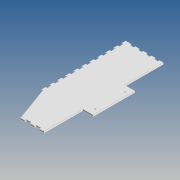
# Autodesk Inventor part: KB33-046-004-008 - Центральная правая боковая пластина
Saved by Autodesk Inventor 2020 (Build 240168000, 168)
## iProperties
Created: 2021-06-25
Part Number: KB33-046-004-008 - Центральная правая боковая пластина
Material: Типовые
Document SubType Name: Modeling
Designer: Петров Иван
Density: 1 g/cm^3
Appearance: По умолчанию
Mass: 112.867 g
Surface Area: 603.849 cm^2
Volume: 112.867 cm^3
Author: Петров Иван
Autodesk Inventor part; units mm, degrees
ref_plane "YZ Plane" through (0, 0, 0) normal (1, 0, 0) x (0, 1, 0)
ref_plane "XZ Plane" through (0, 0, 0) normal (0, 1, 0) x (-1, 0, 0)
ref_plane "XY Plane" through (0, 0, 0) normal (0, 0, 1) x (1, 0, 0)
sketch "Эскиз1" plane through (2.236, 0, -46.8876) normal (0, 1, 0) x (-1, 0, 0)
  line L0 (-10.528, 98.8876) -> (15, 98.8876)
  line L1 (15, 98.8876) -> (15, -5.1124)
  line L2 (15, -5.1124) -> (-10.528, -5.1124)
  line L3 (-10.528, -5.1124) -> (-10.528, 98.8876)
  point P0 (0, 0)
  dimension "d0" = 25.528
  dimension "d1" = 104
  constraints: 8 end point, 2 parallel, 1 horizontal, 1 perpendicular
  measures "d0" distance of L1.end L2.end
  measures "d1" distance of L0.end L1.end
extrude "Выдавливание1" add sketch "Эскиз1" along normal blind 4
sketch "Эскиз2" plane through (2.236, 4, -46.8876) normal (0, 1, 0) x (0, 0, -1)
  circle A0 centre (-9.8876, -0.528) radius 2 projected
  circle A1 centre (-83.8876, -0.528) radius 2 projected
  point P0 (0, 0)
extrude "Выдавливание2" cut sketch "Эскиз2" against normal blind 4
sketch "Эскиз3" plane through (2.236, 4, -46.8876) normal (0, 1, 0) x (1, 0, 0)
  line L0 (-75, -191.6906) -> (-15, -191.6906)
  line L1 (-15, -191.6906) -> (-15, 97.9154)
  line L2 (-15, 97.9154) -> (-75, 97.9154)
  line L3 (-75, 97.9154) -> (-75, -191.6906)
  line L4 (-15, -98.8876) -> (10.528, -98.8876) projected
  line L5 (10.528, 5.1124) -> (-15, 5.1124) projected
  point P0 (-2.236, -46.8876)
  dimension "d8" = 92.803
  dimension "d9" = 92.803
  dimension "d10" = 60
  constraints: 8 end point, 2 parallel, 1 horizontal, 1 perpendicular, 1 point on line
  measures "d8" distance between parallel lines of L4 L0
  measures "d9" distance between parallel lines of L2 L5
  measures "d10" distance between parallel lines of L1 L3
extrude "Выдавливание3" add sketch "Эскиз3" against normal blind 4
sketch "Эскиз4" plane through (2.236, 4, -46.8876) normal (0, 1, 0) x (1, 0, 0)
  line L0 (-75, -191.6906) -> (-75, 97.9154) projected
  line L1 (-75, -191.6906) -> (-105, -109.2663)
  line L2 (-105, -109.2663) -> (-105, 97.9154)
  line L3 (-105, 97.9154) -> (-75, 97.9154)
  line L4 (-2.236, -46.8876) -> (-20.0662, -46.8876)
  dimension "d13" = 30
  dimension "d14" = 90
  dimension "d17" = 20
  constraints: 8 end point, 1 horizontal, 1 parallel
  measures "d13" distance between parallel lines of L0 L2
  measures "d14" angle of L0 L3
  measures "d17" angle of L0 L1
extrude "Выдавливание4" add sketch "Эскиз4" against normal blind 4
sketch "Эскиз5" plane through (-12.764, 0, 144.803) normal (0, 0, 1) x (1, 0, 0)
  line L0 (-60, 4) -> (0, 4) projected
  line L1 (0, 0) -> (-60, 0) projected
  line L2 (-60, 4) -> (-48, 4)
  line L3 (-48, 4) -> (-48, 0)
  line L4 (-48, 0) -> (-60, 0)
  line L5 (-60, 0) -> (-60, 4)
  point P0 (12.764, 0)
  dimension "d18" = 12
  constraints: 8 end point, 2 parallel, 1 horizontal, 1 perpendicular, 1 point on line
  measures "d18" distance of L3.end L4.end
extrude "Выдавливание5" add sketch "Эскиз5" along normal blind 4
pattern_linear "Прямоуг.массив1" count 3 spacing 24 along (1, 0, 0) of "Выдавливание5"
sketch "Эскиз6" plane through (-12.764, 0, -144.803) normal (0, 0, -1) x (-1, 0, 0)
  line L0 (90, 4) -> (60, 4) projected
  line L1 (60, 0) -> (90, 0) projected
  line L2 (90, 4) -> (80, 4)
  line L3 (80, 4) -> (80, 0)
  line L4 (80, 0) -> (90, 0)
  line L5 (90, 0) -> (90, 4)
  point P0 (-12.764, 0)
  point P1 (90, 0)
  point P2 (80, 4)
  dimension "d24" = 10
  constraints: 8 end point, 2 parallel, 1 horizontal, 1 perpendicular, 1 point on line
  measures "d24" distance of L4.end L3.end
extrude "Выдавливание6" add sketch "Эскиз6" along normal blind 4
pattern_linear "Прямоуг.массив2" count 5 spacing 20 along (1, 0, 0) of "Выдавливание6"
sketch "Эскиз7" plane through (2.236, 4, -46.8876) normal (0, 1, 0) x (1, 0, 0)
  line L0 (-105, 101.9154) -> (-105, -109.2663) projected
  line L1 (-105, 101.9154) -> (-109, 101.9154)
  line L2 (-109, 101.9154) -> (-109, 91.9154)
  line L3 (-109, 91.9154) -> (-105, 91.9154)
  line L4 (-105, 91.9154) -> (-105, 101.9154)
  point P0 (-2.236, -46.8876)
  dimension "d30" = 4
  dimension "d31" = 10
  constraints: 8 end point, 2 parallel, 1 horizontal, 1 perpendicular
  measures "d30" distance of L3.end L2.end
  measures "d31" distance of L2.end L1.end
extrude "Выдавливание7" add sketch "Эскиз7" against normal blind 4
pattern_linear "Прямоуг.массив3" count 11 spacing 20 along (0, 0, 1) of "Выдавливание7"
sketch "Эскиз8" plane through (2.236, 0, -46.8876) normal (0, -1, 0) x (1, 0, 0)
  circle A0 centre (-36.9996, -88.3965) radius 2 projected
  circle A1 centre (-36.9996, 182.1718) radius 2 projected
  point P0 (-2.236, 46.8876)
extrude "Выдавливание8" cut sketch "Эскиз8" against normal blind 4
